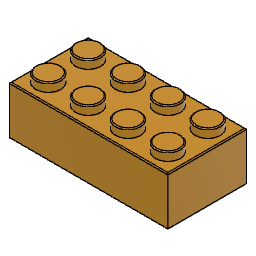
Day #1 - Toy Block v3 (Autodesk Fusion 360 design; units mm, degrees)
Autodesk Fusion 360 part; units mm, degrees
sketch "Sketch1" plane through (0, 0, 0) normal (0, 1, 0) x (1, 0, 0) in component "2x8 Block:1"
  line L0 (0, 0) -> (31.8, 0)
  line L1 (31.8, 0) -> (31.8, 15.8)
  line L2 (31.8, 15.8) -> (0, 15.8)
  line L3 (0, 15.8) -> (0, 0)
  dimension "d1" = 31.8
  dimension "d2" = 15.8
  constraint horizontal L0
  constraint vertical L1
  constraint horizontal L2
  constraint vertical L3
  constraint coincident L0.start L3.end
  measures "d1" distance of L0.start L0.end
  measures "d2" distance of L0.start L2.end
extrude "Extrude1" add sketch "Sketch1" along normal blind 9.6 in component "2x8 Block:1"
sketch "Sketch2" plane through (0, 9.6, 0) normal (0, 1, 0) x (-1, 0, 0) in component "2x8 Block:1"
  line L0 (0, -15.8) -> (0, 0)
  line L1 (0, 0) -> (-31.8, 0)
  line L2 (-31.8, 0) -> (-31.8, -15.8)
  line L3 (-31.8, -15.8) -> (0, -15.8)
  circle A0 centre (-3.9, -11.9) radius 2.5
  dimension "d5" = 5
  dimension "d6" = 3.9
  dimension "d7" = 3.9
  measures "d5" diameter of A0
  measures "d6" distance of L3 A0.centre
  measures "d7" distance of L0 A0.centre
extrude "Extrude2" add sketch "Sketch2" along normal blind 1.7 contours A0 in component "2x8 Block:1"
pattern_linear "R-Pattern1" count 4 spacing 8 along (1, 0, 0) count 2 spacing 8 along (0, 0, 1) of "Extrude2" in component "2x8 Block:1"
shell "Shell1" thickness 1.49 removed faces 1 at (21.2, 0, -5.2667) in component "2x8 Block:1"
sketch "Sketch3" plane through (0, 8.11, 0) normal (0, -1, 0) x (1, 0, 0) in component "2x8 Block:1"
  circle A0 centre (27.9, -3.9) radius 1.01
  circle A1 centre (19.9, -3.9) radius 1.01
  circle A2 centre (11.9, -3.9) radius 1.01
  circle A3 centre (3.9, -3.9) radius 1.01
  circle A4 centre (27.9, -11.9) radius 1.01
  circle A5 centre (19.9, -11.9) radius 1.01
  circle A6 centre (11.9, -11.9) radius 1.01
  circle A7 centre (3.9, -11.9) radius 1.01
  line L0 (1.49, -1.49) -> (1.49, -14.31)
  line L1 (1.49, -14.31) -> (30.31, -14.31)
  line L2 (30.31, -14.31) -> (30.31, -1.49)
  line L3 (30.31, -1.49) -> (1.49, -1.49)
  line L4 (19.9, -11.9) -> (27.9, -3.9) construction
  circle A8 centre (23.9, -7.9) radius 3.15
  circle A9 centre (23.9, -7.9) radius 2.15
  dimension "d15" = 6.3
  dimension "d16" = -1
  constraint coincident A5.centre L4.start
  constraint coincident A0.centre L4.end
  constraint midpoint L4 A8.centre
  measures "d15" diameter of A8
extrude "Extrude3" add sketch "Sketch3" along normal blind 8.1 contours A8 in component "2x8 Block:1"
pattern_linear "R-Pattern2" count 3 spacing 8 along (-1, 0, 0) of "Extrude3" in component "2x8 Block:1"
fillet "Fillet1" radius 0.2 8 edges at (6.2308, 11.3, -4.804) (6.2308, 11.3, -12.804) (14.2308, 11.3, -12.804) (14.2308, 11.3, -4.804) (22.2308, 11.3, -4.804) (22.2308, 11.3, -12.804) (30.2308, 11.3, -4.804) (30.2308, 11.3, -12.804) in component "2x8 Block:1"
fillet "Fillet2" radius 0.2 4 edges at (15.9, 9.6, 0) (0, 9.6, -7.9) (15.9, 9.6, -15.8) (31.8, 9.6, -7.9) in component "2x8 Block:1"
component "2x8 Block:1" placed x (1, 0, 0) y (0, 1, 0) z (0, 0, 1) at (0, 0, 0)
